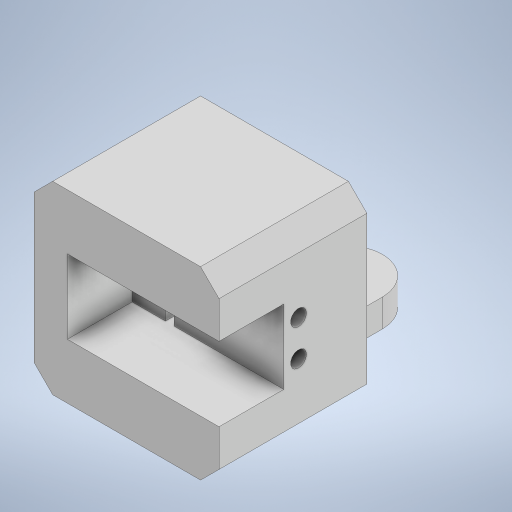
# Autodesk Inventor part: ES117_MP1
Saved by Autodesk Inventor 2024 (Build 280153000, 153)
## iProperties
Created: 2023-06-04
Part Number: ES117_MP1
Material: Generic
Document SubType Name: Modeling
Designer: vilas
Density: 1 g/cm^3
Appearance: Default
Author: vilas
Autodesk Inventor part; units mm, degrees
ref_plane "YZ Plane" through (0, 0, 0) normal (1, 0, 0) x (0, 1, 0)
ref_plane "XZ Plane" through (0, 0, 0) normal (0, 1, 0) x (-1, 0, 0)
ref_plane "XY Plane" through (0, 0, 0) normal (0, 0, 1) x (1, 0, 0)
sketch "Sketch1" plane through (0, 0, 0) normal (0, 0, 1) x (1, 0, 0)
  line L0 (0, 0) -> (50, 0)
  line L1 (50, 0) -> (50, 50)
  line L2 (50, 50) -> (0, 50)
  line L3 (0, 50) -> (0, 0)
  dimension "d0" = 50
  dimension "d1" = 50
  constraints: 8 end point, 2 parallel, 1 horizontal, 1 perpendicular
  measures "d0" distance of L2.end L1.end
  measures "d1" distance of L1.end L0.end
extrude "Extrusion1" add sketch "Sketch1" along normal blind 40
sketch "Sketch2" plane through (0, 0, 40) normal (0, 0, 1) x (1, 0, 0)
  line L0 (50, 0) -> (50, 50) projected
  line L1 (50, 15) -> (9, 15)
  line L2 (9, 15) -> (9, 35)
  line L3 (9, 35) -> (50, 35)
  line L4 (50, 35) -> (50, 15)
  line L5 (0, 0) -> (50, 0) projected
  point P0 (50, 35)
  dimension "d4" = 41
  dimension "d5" = 20
  dimension "d6" = 15
  constraints: 8 end point, 2 parallel, 1 horizontal, 1 perpendicular, 1 point on line
  measures "d4" distance of L2.end L3.end
  measures "d5" distance of L1.end L2.end
  measures "d6" distance between parallel lines of L5 L1
extrude "Extrusion2" cut sketch "Sketch2" against normal blind 17.5
sketch "Sketch3" plane through (0, 0, 0) normal (-1, 0, 0) x (0, 0, 1)
  line L0 (40, 50) -> (40, 0) projected
  line L1 (40, 35) -> (18.5, 35) construction
  line L2 (40, 35) -> (61.5, 35) construction
  line L3 (18.5, 35) -> (18.5, 15) construction
  line L4 (18.5, 15) -> (40, 15) construction
  line L5 (0, 50) -> (40, 50) projected
  line L6 (40, 29.85) -> (18.5, 29.85) construction
  line L7 (40, 20.15) -> (18.5, 20.15) construction
  point P0 (0, 0)
  dimension "d9" = 21.5
  dimension "d10" = 180
  dimension "d11" = 20
  dimension "d12" = 15
  dimension "d13" = 5.15
  dimension "d14" = 5.15
  constraints: 12 end point, 6 point on line, 3 horizontal, 3 perpendicular, 1 collinear
  measures "d9" distance of L1.start L1.end
  measures "d10" angle of L1 L2
  measures "d11" distance of L1.end L3.end
  measures "d12" distance between parallel lines of L5 L1
  measures "d13" distance between parallel lines of L6 L1
  measures "d14" distance between parallel lines of L4 L7
hole "Hole1" at (0, 29.85, 18.5) at (0, 20.15, 18.5) direction (1, 0, 0) diameter 4.3 end through all
sketch "Sketch4" plane through (0, 0, 22.5) normal (0, 0, 1) x (1, 0, 0)
  line L0 (9, 35) -> (50, 35) projected
  line L1 (50, 15) -> (9, 15) projected
  line L2 (18, 35) -> (20.4, 35)
  line L3 (20.4, 35) -> (20.4, 15)
  line L4 (20.4, 15) -> (18, 15)
  line L5 (18, 15) -> (18, 35)
  line L6 (9, 15) -> (9, 35) projected
  point P0 (0, 0)
  point P1 (18, 15)
  dimension "d22" = 9
  dimension "d23" = 2.4
  constraints: 8 end point, 2 parallel, 2 point on line, 1 horizontal, 1 perpendicular
  measures "d22" distance between parallel lines of L5 L6
  measures "d23" distance between parallel lines of L3 L5
extrude "Extrusion3" cut sketch "Sketch4" against normal blind 7 contours L0 L3 L1 L5
chamfer "Chamfer1" distance 5 angle 45 4 edges at (0, 50, 20) (50, 50, 20) (0, 0, 20) (50, 0, 20)
sketch "Sketch7" plane through (0, 0, 22.5) normal (0, 0, 1) x (1, 0, 0)
  line L0 (18, 15) -> (18, 35) projected
  line L1 (18, 24.5) -> (16, 24.5)
  line L2 (16, 24.5) -> (16, 25.5)
  line L3 (16, 25.5) -> (18, 25.5)
  line L4 (18, 25.5) -> (18, 24.5)
  line L5 (9, 35) -> (50, 35) projected
  point P0 (0, 0)
  dimension "d45" = 2
  dimension "d46" = 1
  dimension "d47" = 9.5
  constraints: 8 end point, 2 parallel, 1 horizontal, 1 perpendicular, 1 point on line
  measures "d45" distance of L2.end L3.end
  measures "d46" distance of L1.end L2.end
  measures "d47" distance between parallel lines of L3 L5
extrude "Extrusion5" cut sketch "Sketch7" against normal blind 7
chamfer "Chamfer3" distance 7 distance2 2 1 edges at (16, 25, 15.5) measured on face at (16, 25.1667, 20.1667)
sketch "Sketch8" plane through (0, 0, 0) normal (0, 0, -1) x (-1, 0, 0)
  line L0 (-5, 0) -> (-45, 0) projected
  line L1 (-14.2086, 0) -> (-34.2086, 0)
  line L2 (-34.2086, 0) -> (-34.2086, 7.5)
  line L3 (-34.2086, 7.5) -> (-14.2086, 7.5)
  line L4 (-14.2086, 7.5) -> (-14.2086, 0)
  point P0 (0, 0)
  dimension "d53" = 20
  dimension "d54" = 7.5
  constraints: 8 end point, 2 parallel, 1 horizontal, 1 perpendicular, 1 point on line
  measures "d53" distance of L2.end L3.end
  measures "d54" distance of L1.end L2.end
extrude "Extrusion6" add sketch "Sketch8" along normal blind 30
fillet "Fillet2" radius 10 2 edges at (34.2086, 3.75, -30) (14.2086, 3.75, -30)
chamfer "Chamfer4" distance 3 angle 45 2 edges at (34.2086, 3.75, 0) (14.2086, 3.75, 0)
sketch "Sketch9" plane through (24.2086, 7.5, -20) normal (0, 1, 0) x (1, 0, 0)
  line L0 (13, -20) -> (-13, -20) projected
  line L1 (0, -20) -> (0, 0) construction
  point P0 (-24.2086, -20)
  dimension "d61" = 20
  constraints: 2 end point, 1 midpoint, 1 vertical
  measures "d61" distance of L1.start L1.end
hole "Hole3" at (24.2086, 7.5, -20) direction (0, -1, 0) diameter 5 end through all counterbore diameter 6 counterbore depth 4
body "Solid1"
